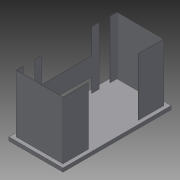
# Autodesk Inventor part: soccer_goal.ipj
Saved by Autodesk Inventor 2015 SP1 (Build 190203100, 203)
## iProperties
Created: 2018-04-10
Part Number: soccer_goal.ipj
Material: Generic
Document SubType Name: Modeling
Designer: 407642
Density: 1 g/cm^3
Appearance: Default
Author: 407642
Autodesk Inventor part; units mm, degrees
ref_plane "YZ Plane" through (0, 0, 0) normal (1, 0, 0) x (0, 1, 0)
ref_plane "XZ Plane" through (0, 0, 0) normal (0, 1, 0) x (-1, 0, 0)
ref_plane "XY Plane" through (0, 0, 0) normal (0, 0, 1) x (1, 0, 0)
sketch "Sketch1" plane through (0, 0, 0) normal (0, 1, 0) x (-1, 0, 0)
  line L0 (0, 213.3361) -> (190.5, 213.3361)
  line L1 (190.5, 213.3361) -> (190.5, -167.6639)
  line L2 (190.5, -167.6639) -> (0, -167.6639)
  line L3 (0, -167.6639) -> (0, 213.3361)
  point P0 (0, 0)
  dimension "d0" = 190.5
  dimension "d1" = 381
  constraints: 8 end point, 2 parallel, 1 horizontal, 1 perpendicular
  measures "d0" distance of L1.end L2.end
  measures "d1" distance of L0.end L1.end
extrude "Extrusion1" add sketch "Sketch1" along normal blind 12.7
sketch "Sketch2" plane through (0, 12.7, 0) normal (0, 1, 0) x (1, 0, 0)
  line L0 (0, -213.3361) -> (-190.5, -213.3361)
  line L1 (-190.5, -213.3361) -> (-190.5, 167.6639)
  line L2 (-190.5, 167.6639) -> (0, 167.6639)
  line L3 (0, 167.6639) -> (0, -213.3361)
  line L4 (-177.8, 154.9639) -> (-177.8, -200.6361)
  line L5 (-177.8, -200.6361) -> (-12.7, -200.6361)
  line L6 (-12.7, -200.6361) -> (-12.7, 154.9639)
  line L7 (-12.7, 154.9639) -> (-177.8, 154.9639)
  line L8 (-177.0062, -199.8424) -> (-177.0062, 154.1701)
  line L9 (-177.0062, 154.1701) -> (-13.4938, 154.1701)
  line L10 (-13.4938, 154.1701) -> (-13.4938, -199.8424)
  line L11 (-13.4938, -199.8424) -> (-177.0062, -199.8424)
  point P0 (0, 0)
  dimension "d4" = 12.7
  dimension "d5" = 0.7937
  constraints: 24 end point, 6 parallel, 3 perpendicular, 1 horizontal, 6 other
  measures "d4" distance between parallel lines of L1 L4
  measures "d5" distance between parallel lines of L4 L8
extrude "Extrusion2" add sketch "Sketch2" along normal blind 203.2 contours L7 L6 L5 L4
sketch "Sketch3" plane through (-12.7, 12.7, 200.6361) normal (1, 0, 0) x (0, 0, -1)
  line L0 (354.8062, 203.2) -> (265.9062, 203.2)
  line L1 (265.9062, 203.2) -> (265.9062, 0)
  line L2 (265.9062, 0) -> (354.8062, 0)
  line L3 (354.8062, 0) -> (354.8062, 203.2)
  line L4 (354.8062, 0) -> (0.7938, 0) projected
  line L5 (0.7938, 203.2) -> (89.6938, 203.2)
  line L6 (89.6938, 203.2) -> (89.6938, 0)
  line L7 (89.6938, 0) -> (0.7938, 0)
  line L8 (0.7938, 0) -> (0.7938, 203.2)
  line L9 (89.6938, 203.2) -> (265.9062, 203.2)
  line L10 (265.9062, 203.2) -> (265.9062, 0)
  line L11 (265.9062, 0) -> (89.6938, 0)
  line L12 (89.6938, 0) -> (89.6938, 203.2)
  point P0 (200.6361, -12.7)
  point P1 (0, 203.2)
  dimension "d9" = 88.9
  dimension "d10" = 88.9
  constraints: 24 end point, 6 parallel, 3 horizontal, 3 perpendicular, 1 point on line
  measures "d9" distance of L2.end L1.end
  measures "d10" distance of L6.end L7.end
extrude "Extrusion3" cut sketch "Sketch3" against normal blind 50.8 contours L1 L4 L6 L9
sketch "Sketch4" plane through (-177.0062, 12.7, 199.8424) normal (1, 0, 0) x (0, 0, -1)
  line L0 (265.1125, 0) -> (265.1125, 203.2) projected
  line L1 (88.9, 0) -> (265.1125, 0)
  line L2 (265.1125, 0) -> (265.1125, 50.8)
  line L3 (265.1125, 50.8) -> (88.9, 50.8)
  line L4 (88.9, 50.8) -> (88.9, 0)
  line L5 (88.9, 203.2) -> (265.1125, 203.2)
  line L6 (265.1125, 203.2) -> (265.1125, 114.3)
  line L7 (265.1125, 114.3) -> (88.9, 114.3)
  line L8 (88.9, 114.3) -> (88.9, 203.2)
  point P0 (199.8424, -12.7)
  dimension "d13" = 50.8
  dimension "d14" = 88.9
  constraints: 16 end point, 4 parallel, 2 horizontal, 2 perpendicular, 2 point on line
  measures "d13" distance of L2.end L1.end
  measures "d14" distance of L5.end L6.end
extrude "Extrusion4" cut sketch "Sketch4" against normal blind 50.8
sketch "Sketch5" plane through (-177.8, 12.7, 200.6361) normal (-1, 0, 0) x (0, 0, 1)
  line L0 (-265.9062, 114.3) -> (-265.9062, 203.2) projected
  line L1 (-355.6, 0) -> (-355.6, 203.2) projected
  line L2 (-368.3, 0) -> (12.7, 0) projected
  line L3 (-355.6, 203.2) -> (-330.2, 203.2)
  line L4 (-330.2, 203.2) -> (-330.2, 0)
  line L5 (-330.2, 0) -> (-355.6, 0)
  line L6 (-355.6, 0) -> (-355.6, 203.2)
  line L7 (-265.9062, 203.2) -> (-291.3062, 203.2)
  line L8 (-291.3062, 203.2) -> (-291.3062, 0)
  line L9 (-291.3062, 0) -> (-265.9062, 0)
  line L10 (-265.9062, 0) -> (-265.9062, 203.2)
  line L11 (-330.2, 203.2) -> (-291.3062, 203.2)
  line L12 (-291.3062, 203.2) -> (-291.3062, 0)
  line L13 (-291.3062, 0) -> (-330.2, 0)
  line L14 (-330.2, 0) -> (-330.2, 203.2)
  point P0 (-200.6361, -12.7)
  dimension "d17" = 89.6937
  dimension "d18" = 25.4
  dimension "d19" = 25.4
  constraints: 24 end point, 6 parallel, 3 horizontal, 3 perpendicular, 2 point on line
  measures "d17" distance between parallel lines of L0 L1
  measures "d18" distance of L4.end L5.end
  measures "d19" distance of L9.end L8.end
extrude "Extrusion5" cut sketch "Sketch5" against normal blind 25.4 contours L8 L2 L4 L11
sketch "Sketch6" plane through (-177.8, 12.7, 200.6361) normal (-1, 0, 0) x (0, 0, 1)
  line L0 (-89.6938, 114.3) -> (-265.9062, 114.3) projected
  line L1 (0, 0) -> (-89.6938, 0) projected
  line L2 (0, 203.2) -> (-25.4, 203.2)
  line L3 (-25.4, 203.2) -> (-25.4, 0)
  line L4 (-25.4, 0) -> (0, 0)
  line L5 (0, 0) -> (0, 203.2)
  line L6 (-89.6938, 203.2) -> (0, 203.2) projected
  line L7 (-89.6938, 0) -> (-64.2938, 0)
  line L8 (-64.2938, 0) -> (-64.2938, 203.2)
  line L9 (-64.2938, 203.2) -> (-89.6938, 203.2)
  line L10 (-89.6938, 203.2) -> (-89.6938, 0)
  line L11 (-64.2938, 203.2) -> (-25.4, 203.2)
  line L12 (-25.4, 203.2) -> (-25.4, 0)
  line L13 (-25.4, 0) -> (-64.2938, 0)
  line L14 (-64.2938, 0) -> (-64.2938, 203.2)
  line L15 (-64.2938, 203.2) -> (-25.4, 203.2)
  line L16 (-25.4, 203.2) -> (-25.4, 0)
  line L17 (-25.4, 0) -> (-64.2938, 0)
  line L18 (-64.2938, 0) -> (-64.2938, 203.2)
  point P0 (-200.6361, -12.7)
  dimension "d22" = 25.4
  dimension "d23" = 25.4
  constraints: 32 end point, 8 parallel, 4 horizontal, 4 perpendicular, 2 point on line
  measures "d22" distance of L4.end L3.end
  measures "d23" distance of L9.end L8.end
extrude "Extrusion6" cut sketch "Sketch6" against normal blind 25.4 contours L1 L8 L6 L3
body "Solid1"
